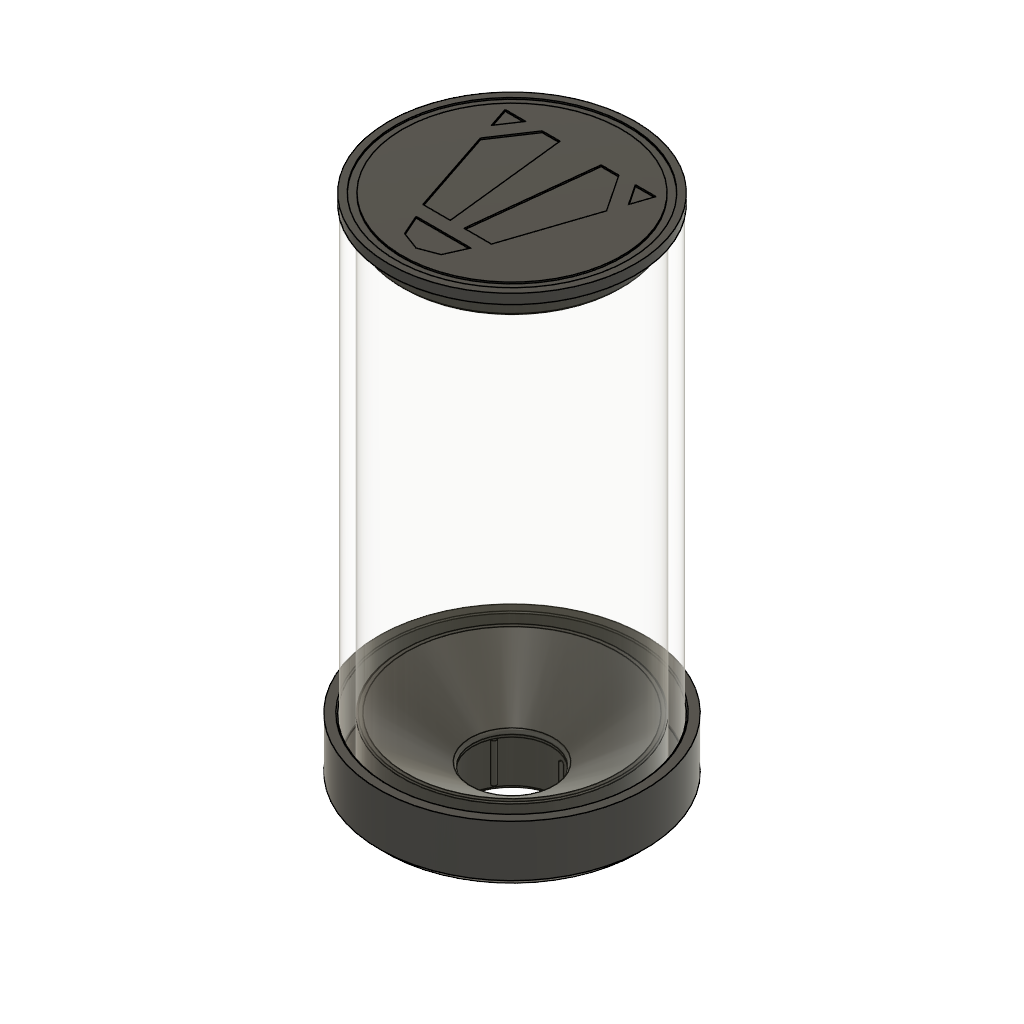
Trickler (Autodesk Fusion 360 archive; units mm, degrees)
design "PowderContainer"
part number: 2026-04-14-16-20-41-609
Autodesk Fusion 360 part; units mm, degrees
note: some values were not read from the file. Chosen so that the rebuilt part matches the saved one: how an offset face is resized. Set by a fixed rule: which sketch regions a step uses.
sketch "Sketch1" plane through (0, 0, 0) normal (0, 1, 0) x (1, 0, 0)
  circle A0 centre (0, 0) radius 25
  circle A1 centre (0, 0) radius 22.65
  dimension "d1" = 50
  dimension "d2" = 45.3
  constraint coincident A0.centre A1.centre
  measures "d1" diameter of A0
  measures "d2" diameter of A1
extrude "Extrude1" add sketch "Sketch1" along normal blind 100 makes body 1
sketch "Sketch2" plane through (0, 0, 0) normal (0, 1, 0) x (1, 0, 0)
  circle A0 centre (0, 0) radius 22.5
  circle A1 centre (0, 0) radius 25.2
  circle A2 centre (0, 0) radius 10.05
  circle A3 centre (0, 0) radius 12.05
  circle A4 centre (0, 0) radius 27.2
  circle A5 centre (0, 0) radius 8.05
  line L0 (0, -10.05) -> (8.7036, 5.025)
  line L1 (8.7036, 5.025) -> (-8.7036, 5.025)
  line L2 (-8.7036, 5.025) -> (0, -10.05)
  circle A6 centre (0, -10.05) radius 0.5
  circle A7 centre (8.7036, 5.025) radius 0.5
  circle A8 centre (-8.7036, 5.025) radius 0.5
  circle A9 centre (0, 0) radius 21
  dimension "d5" = 45
  dimension "d6" = 50.4
  dimension "d7" = 20.1
  dimension "d8" = 24.1
  dimension "d9" = 54.4
  dimension "d14" = 16.1
  dimension "d31" = 10.05
  dimension "d32" = 1
  dimension "d33" = 1
  dimension "d34" = 1
  dimension "d51" = 42
  constraint coincident A0.centre A1.centre
  constraint concentric A0 A1
  constraint concentric A1 A2
  constraint concentric A2 A3
  constraint concentric A0 A4
  constraint concentric A0 A5
  constraint coincident L0.start L2.end
  constraint coincident L0.end L1.start
  constraint coincident L1.end L2.start
  constraint concentric A2 A9
  measures "d5" diameter of A0
  measures "d6" diameter of A1
  measures "d7" diameter of A2
  measures "d8" diameter of A3
  measures "d9" diameter of A4
  measures "d14" diameter of A5
  measures "d31" distance of L0.start A0.centre
  measures "d32" diameter of A6
  measures "d33" diameter of A7
  measures "d34" diameter of A8
  measures "d51" diameter of A9
extrude "Extrude2" add sketch "Sketch2" along normal blind 10 separate body contours A0 | A2 A7 | A2 A6 | A2 A8 | A3 | A4 | A9 makes body 2 at (27.1662, 6.6667, 1.3558) makes body 3 at (22.472, 6.6667, 1.1215)
extrude "Extrude3" add sketch "Sketch2" against normal blind 2 contours A0 | A1 | A2 A7 | A2 A6 | A2 A8 | A3 | A4 | A9 bodies 2 3
extrude "Extrude4" add sketch "Sketch2" along normal blind 10 contours A2 A5 L0 A6 A7 | A2 L0 A7 | A2 L0 A6 | A2 L1 A7 | L0 L1 A7 | A5 L0 L1 A7 | L0 L2 A6 | A2 L2 A6 | A5 L0 L2 A6 | A2 A5 L1 A7 A8 | A2 A5 L2 A6 A8 | A2 L1 A8 | A2 L2 A8 | L1 L2 A8 | A5 L1 L2 A8 bodies 2
extrude "Extrude5" add sketch "Sketch2" against normal blind 11 contours A2 A7 | A2 A6 | A2 A8 | A3 bodies 2
chamfer "Chamfer4" distance 0.25 angle 45 2 edges at (-20.9774, 10, 8.1363) (-23.4946, 10, -9.1127) on bodies 2
chamfer "Chamfer5" distance 1.5 angle 45 1 edges at (-25.3593, -2, -9.8359) on bodies 2
chamfer "Chamfer6" distance 2 distance2 9 1 edges at (-11.2345, -2, 4.3575) measured on face at (21.0095, -2, 1.8754) on bodies 2
chamfer "Chamfer7" distance 1.5 angle 45 1 edges at (-13.0992, -2, -5.0807) on bodies 2
chamfer "Chamfer8" distance 13.5 distance2 9 1 edges at (-7.5052, 10, -2.911) measured on face at (17.4039, 10, 1.5053) on bodies 2
chamfer "Chamfer9" distance 0.5 distance2 0.5 1 edges at (-9.3699, 0, 3.6342) measured on face at (10.0375, -7.3333, 0.501) on bodies 2
extrude "Extrude7" add sketch "Sketch2" along normal blind -10 and the other way blind 1 contours A2 L0 A7 | A2 L0 A6 | A2 L1 A7 | L0 L1 A7 | L0 L2 A6 | A2 L2 A6 | A2 L1 A8 | A2 L2 A8 | L1 L2 A8 bodies 2
chamfer "Chamfer10" distance 0.5 angle 45 6 edges at (-8.2705, -1, -4.775) (-8.2705, -10, -4.775) (8.2705, -10, -4.775) (8.2705, -1, -4.775) (0, -1, 9.55) (0, -10, 9.55) on bodies 2
fillet "Fillet1" radius 1 1 edges at (-7.5052, 1, -2.911) on bodies 2
chamfer "Chamfer11" distance 1 angle 45 1 edges at (-9.3699, -11, 3.6342) on bodies 2
extrude "Extrude8" add sketch "Sketch2" along normal blind 100 and the other way blind -102 separate body contours A0 | A1 | A2 A5 L0 A6 A7 | A2 L0 A7 | A2 A7 | A2 A6 | A2 L0 A6 | A2 L1 A7 | L0 L1 A7 | A5 L0 L1 A7 | L0 L2 A6 | A2 L2 A6 | A5 L0 L2 A6 | A2 A5 L1 A7 A8 | A5 L0 L1 L2 | A5 L0 | A2 A5 L2 A6 A8 | A2 L1 A8 | A2 A8 | A5 L1 | A2 L2 A8 | A5 L2 | L1 L2 A8 | A5 L1 L2 A8 | A3 | A9 makes body 4
extrude "Extrude9" add sketch "Sketch2" along normal blind 100 and the other way blind -96 contours A0 bodies 4
chamfer "Chamfer12" distance 0.5 angle 45 1 edges at (-20.9774, 96, 8.1363) on bodies 4
sketch "Sketch3" plane through (0, 0, 0) normal (0, 0, 1) x (1, 0, 0)
  line L0 (0, 0) -> (0, -11)
  line L1 (0.5, -11) -> (-0.5, -11)
  line L2 (-0.5, -11) -> (-0.5, 0)
  line L3 (-0.5, 0) -> (0.5, 0)
  line L4 (0.5, 0) -> (0.5, -11)
  line L5 (0.5, -11) -> (-0.5, 0) construction
  line L6 (-0.5, -11) -> (0.5, 0) construction
  line L7 (0, 0) -> (0, -4)
  circle A0 centre (0, -4) radius 0.5
  point P0 (0, -5.5)
  dimension "d61" = 11
  dimension "d62" = 1
  dimension "d63" = 11
  dimension "d64" = 4
  dimension "d65" = 1
  constraint coincident L0.start L7.start
  constraint vertical L0
  constraint horizontal L1
  constraint perpendicular L1 L2
  constraint parallel L1 L3
  constraint parallel L2 L4
  constraint coincident L5 P0
  constraint coincident L6 P0
  constraint midpoint L0 P0
  constraint perpendicular L3 L7
  constraint coincident L7.end A0.centre
  measures "d61" distance of L0.start L0.end
  measures "d62" distance of L2.end L3.end
  measures "d63" distance of L1.end L2.end
  measures "d64" distance of L0.start L7.end
  measures "d65" diameter of A0
extrude "Extrude10" cut sketch "Sketch3" against normal blind 26 contours L0 L7 A0 | L0 L7 A0 | L0 L1 L4 A0 | L0 L1 L2 A0 bodies 2
sketch "Logo" plane through (0, 102, 0) normal (0, 1, 0) x (1, 0, 0)
  line L0 (-7.8348, 14) -> (-10.2703, 10.3468)
  line L1 (-1.4, -11.2) -> (-4.2, 14)
  line L2 (-12.8783, 6.4348) -> (-7, -11.2)
  line L3 (-4.2, 14) -> (-7.8348, 14)
  line L4 (-7, -11.2) -> (-1.4, -11.2)
  line L5 (-10.2703, 10.3468) -> (-12.8783, 6.4348)
  line L6 (7.8348, 14) -> (4.2, 14)
  line L7 (12.8783, 6.4348) -> (10.2703, 10.3468)
  line L8 (1.4, -11.2) -> (7, -11.2)
  line L9 (4.2, 14) -> (1.4, -11.2)
  line L10 (10.2703, 10.3468) -> (7.8348, 14)
  line L11 (7, -11.2) -> (12.8783, 6.4348)
  line L12 (5.6, -14) -> (3.7333, -18.2)
  line L13 (-3.7333, -18.2) -> (-5.6, -14)
  line L14 (0, -19.6) -> (-3.7333, -18.2)
  line L15 (-5.6, -14) -> (5.6, -14)
  line L16 (3.7333, -18.2) -> (0, -19.6)
  circle A0 centre (0, 0) radius 22.4
  circle A1 centre (0, 0) radius 23.8
  line L17 (-14, 9.8) -> (-15.4, 14)
  line L18 (-15.4, 14) -> (-11.2, 14)
  line L19 (-11.2, 14) -> (-14, 9.8)
  line L20 (14, 9.8) -> (11.2, 14)
  line L21 (11.2, 14) -> (15.4, 14)
  line L22 (15.4, 14) -> (14, 9.8)
scale "Scale1" [no effect]
extrude "Extrude11" cut sketch "Logo" against normal blind 0.3 bodies 4
equation "d2 = d1 - ( ( 2.35 * 2 ) * 1 mm )"
equation "d5 = d2 - 0.3 mm"
equation "d6 = d1 + 0.40 mm"
equation "d8 = d7 + 4 mm"
equation "d9 = d6 + 4 mm"
equation "d14 = d7 - 4 mm"
equation "d31 = d7 / 2"
equation "d33 = d32"
equation "d34 = d32"
equation "d51 = d5 - 3 mm"
equation "d63 = d61"
equation "d65 = d62"
named bodies: "Acrylic Pipe", "ReservoirAdapter", "ReservoirCap"

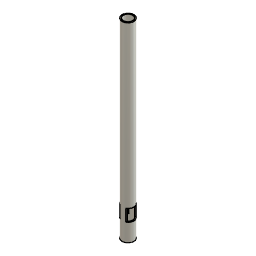
design "Pipe"
part number: 2026-04-14-16-00-10-104
Autodesk Fusion 360 part; units mm, degrees
sketch "Sketch1" plane through (0, 0, 0) normal (0, 1, 0) x (1, 0, 0)
  circle A0 centre (0, 0) radius 5
  circle A1 centre (0, 0) radius 4
  dimension "d1" = 10
  dimension "d2" = 8
  constraint coincident A0.centre A1.centre
  measures "d1" diameter of A0
  measures "d2" diameter of A1
extrude "Extrude1" add sketch "Sketch1" along normal blind 160
sketch "Sketch2" plane through (0, 0, 0) normal (0, 0, 1) x (1, 0, 0)
  line L0 (-5, 0) -> (5, 0)
  line L1 (5, 0) -> (5, 15)
  line L2 (5, 15) -> (-5, 15)
  line L3 (-5, 15) -> (-5, 0)
  line L4 (-5, 15) -> (5, 15)
  line L5 (5, 15) -> (5, 25)
  line L6 (5, 25) -> (-5, 25)
  line L7 (-5, 25) -> (-5, 15)
  line L8 (-5, 25) -> (-2.5, 25)
  line L9 (-2.5, 25) -> (-2.5, 15)
  line L10 (-2.5, 15) -> (-5, 15)
  line L11 (-5, 15) -> (-5, 25)
  line L12 (5, 15) -> (2.5, 15)
  line L13 (2.5, 15) -> (2.5, 25)
  line L14 (2.5, 25) -> (5, 25)
  line L15 (5, 25) -> (5, 15)
  dimension "d5" = 10
  dimension "d6" = 15
  dimension "d7" = 10
  dimension "d8" = 10
  dimension "d9" = 2.5
  dimension "d10" = 10
  dimension "d11" = 2.5
  dimension "d12" = 10
  constraint horizontal L0
  constraint vertical L1
  constraint horizontal L2
  constraint vertical L3
  constraint horizontal L4
  constraint vertical L5
  constraint horizontal L6
  constraint vertical L7
  constraint horizontal L8
  constraint vertical L9
  constraint horizontal L10
  constraint vertical L11
  constraint horizontal L12
  constraint vertical L13
  constraint horizontal L14
  constraint vertical L15
  measures "d5" distance of L0.start L0.end
  measures "d6" distance of L0.start L2.end
  measures "d7" distance of L2.end L1.end
  measures "d8" distance of L2.end L6.end
  measures "d9" distance of L6.end L8.end
  measures "d10" distance of L6.end L2.end
  measures "d11" distance of L1.end L12.end
  measures "d12" distance of L1.end L5.end
extrude "Extrude2" cut sketch "Sketch2" along normal mid plane 20 contours L2 L4 L6 L7 L8 L9 L10 L11 | L2 L4 L5 L6 L12 L13 L14 L15
equation "d2 = d1 - 2 mm"
equation "d5 = d1"
equation "d7 = d1"
equation "d9 = d1 / 4"
equation "d10 = d1"
equation "d11 = d1 / 4"
equation "d12 = d1"
equation "d13 = d1"
named bodies: "Pipe"

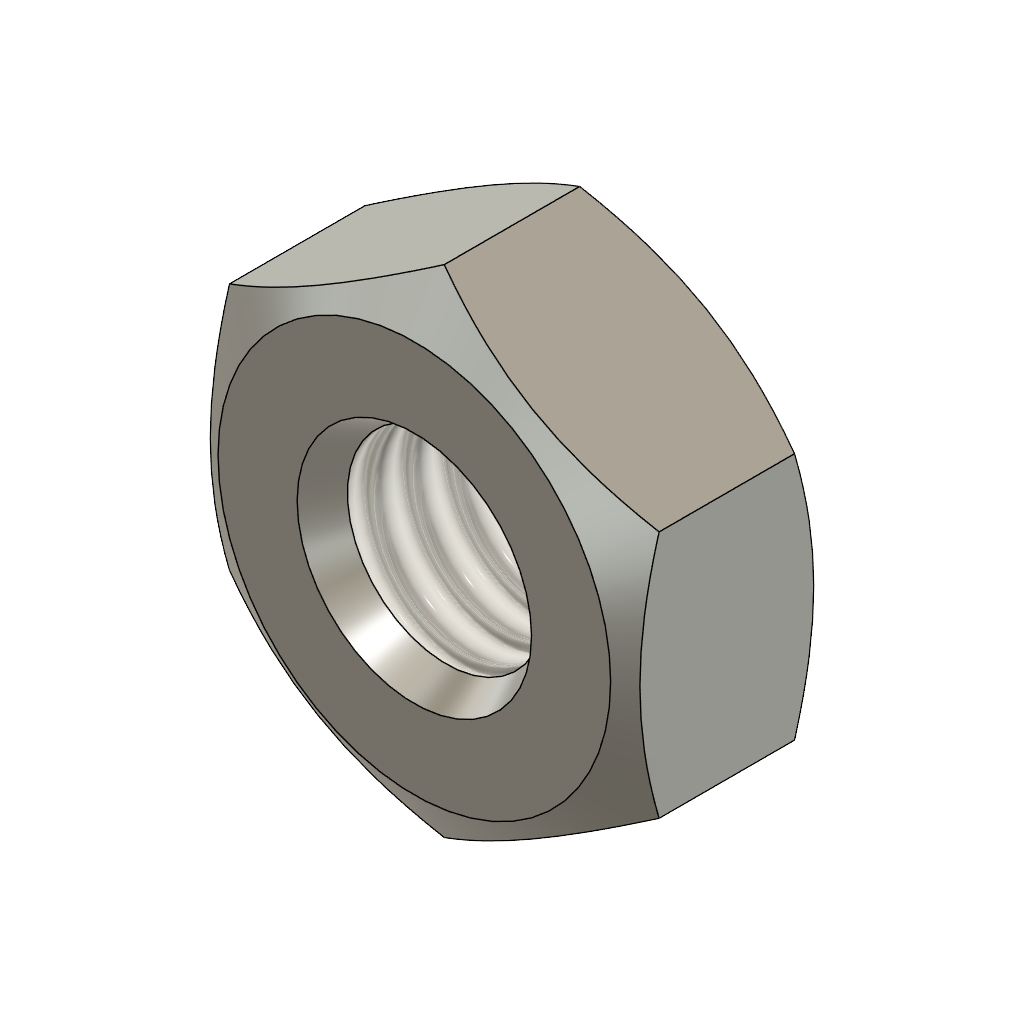
design "Hexagon Nut DIN EN 14399-4 - M3 Steel 6 Plain"
description: Hexagon Nut DIN EN 14399-4 - M3
part number: DIN EN 14399-4 - M3 Steel 6 Plain
Autodesk Fusion 360 part; units mm, degrees
sketch "Sketch1" plane through (0, 0, 0) normal (0, 1, 0) x (1, 0, 0)
  line L0 (0, 0) -> (0, -2.5)
  line L1 (-1.5, 0) -> (-2.5125, 0)
  line L2 (-2.5125, 0) -> (-3.1762, -0.3832)
  line L3 (-3.1762, -0.3832) -> (-3.1762, -2.1168)
  line L4 (-3.1762, -2.1168) -> (-2.5125, -2.5)
  line L5 (-2.5125, -2.5) -> (-1.5, -2.5)
  line L6 (-1.5, -2.5) -> (-1.5, 0)
  dimension "d121" = 3
  dimension "d122" = 30
  dimension "d123" = 30
  dimension "d128" = 6.3525
  dimension "d172" = 5.025
  dimension "d179" = 2.5
  constraint vertical L0
  constraint coincident L0 L0.end
  constraint coincident origin L0
  constraint horizontal L1
  constraint coincident L0.start L1
  constraint coincident L0.start origin
  constraint coincident L0.end L5
  constraint vertical L1.end L4.end
  measures "d122" angle of L1 L2
  measures "d123" angle of L4 L5
  measures "d179" distance of L1 L5
revolve "Revolve1" add sketch "Sketch1" angle 360 about axis through (0, 0, 0) along (0, 0, 1)
sketch "Sketch8" plane through (0, 0, 2.5) normal (0, 0, 1) x (1, 0, 0)
  line L0 (-2.75, -1.5894) -> (-2.75, 1.5894)
  circle A0 centre (0, 0) radius 1.5
  circle A1 centre (0, 0) radius 3.1762
  dimension "d114" = 2.75
  constraint coincident L0.end A1
  constraint coincident L0.start A1
  constraint vertical L0
  measures "d114" distance of A0.centre L0
extrude "Extrude5" cut sketch "Sketch8" against normal blind 2.5 contours L0 A1 picked at (-2.8188, -0.3871)
pattern_circular "C-Pattern2" count 6 over 360 about axis through (0, 0, 1.75) along (0, 0, 1) of "Extrude5"
thread "Thread3" "ISO Metric profile 3.0 M3x0.5 M3x0.5 6H" major diameter 3.086 minor diameter 2.529 pitch 0.5 angle 60 resizes the face on face at (-1.4981, 0.0748, 1.6667)
sketch "Sketch12" plane through (0, 0, 0) normal (0, 1, 0) x (1, 0, 0)
  line L0 (-1.5, 0) -> (0, 0)
  line L1 (-0.7783, -1.25) -> (-1.5, 0)
  line L2 (-1.5, -2.5) -> (0, -2.5)
  line L3 (-0.7783, -1.25) -> (-1.5, -2.5)
  line L4 (0, 0) -> (0, -2.5)
  dimension "d169" = 60
  dimension "d177" = 1.5
  dimension "d178" = 60
  constraint horizontal L0
  constraint coincident L1.start L3.start
  constraint vertical L0.start L2.start
  constraint coincident L2.end L4.end
  constraint coincident L0.end L4.start
  constraint perpendicular L2 L4
  measures "d169" angle of L2 L3
  measures "d177" distance of L0.start L4
  measures "d178" angle of L0 L1
revolve "Revolve3" cut sketch "Sketch12" angle 360 about axis through (0, 0, 1.75) along (0, 0, 1)
equation "adsk_nheig = 2.50 mm"
equation "adsk_maxdia = 6.3525 mm"
equation "adsk_nomdia = 3.00 mm"
equation "d89 = -adsk_nheig"
equation "adsk_waflat = 5.50 mm"
equation "d114 = adsk_waflat / 2"
equation "adsk_chamang1 = 30.00 deg"
equation "adsk_chamang2 = 30.00 deg"
equation "d121 = adsk_nomdia"
equation "d122 = adsk_chamang1"
equation "d123 = adsk_chamang2"
equation "d128 = adsk_maxdia"
equation "d163 = adsk_nheig"
equation "adsk_beardia = 5.025 mm"
equation "d172 = adsk_beardia"
equation "d177 = adsk_nomdia * 0.5"
equation "d179 = adsk_nheig"

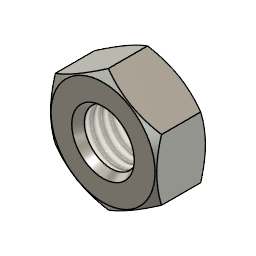
design "Hexagon Nut DIN 934 - M10 x 1.5 Steel 6 Plain"
description: Hexagon Nut DIN 934 - M10 x 1.5
part number: DIN 934 - M10 x 1.5 Steel 6 Plain
Autodesk Fusion 360 part; units mm, degrees
sketch "Sketch1" plane through (0, 0, 0) normal (0, 1, 0) x (1, 0, 0)
  line L0 (0, 0) -> (0, -8)
  line L1 (-5, 0) -> (-8.33, 0)
  line L2 (-8.33, 0) -> (-9.8175, -0.8588)
  line L3 (-9.8175, -0.8588) -> (-9.8175, -7.1412)
  line L4 (-9.8175, -7.1412) -> (-8.33, -8)
  line L5 (-8.33, -8) -> (-5, -8)
  line L6 (-5, -8) -> (-5, 0)
  dimension "d121" = 10
  dimension "d122" = 30
  dimension "d123" = 30
  dimension "d128" = 19.635
  dimension "d172" = 16.66
  dimension "d179" = 8
  constraint vertical L0
  constraint coincident L0 L0.end
  constraint coincident origin L0
  constraint horizontal L1
  constraint coincident L0.start L1
  constraint coincident L0.start origin
  constraint coincident L0.end L5
  constraint vertical L1.end L4.end
  measures "d122" angle of L1 L2
  measures "d123" angle of L4 L5
  measures "d179" distance of L1 L5
revolve "Revolve1" add sketch "Sketch1" angle 360 about axis through (0, 0, 0) along (0, 0, 1)
sketch "Sketch8" plane through (0, 0, 8) normal (0, 0, 1) x (1, 0, 0)
  line L0 (-8.5, -4.9126) -> (-8.5, 4.9126)
  circle A0 centre (0, 0) radius 5
  circle A1 centre (0, 0) radius 9.8175
  dimension "d114" = 8.5
  constraint coincident L0.end A1
  constraint coincident L0.start A1
  constraint vertical L0
  measures "d114" distance of A0.centre L0
extrude "Extrude5" cut sketch "Sketch8" against normal blind 8 contours L0 A1 picked at (-8.7126, 1.1966)
pattern_circular "C-Pattern2" count 6 over 360 about axis through (0, 0, 1.75) along (0, 0, 1) of "Extrude5"
thread "Thread3" "ISO Metric profile 10.0 M10x1.5 M10x1.5 6H" major diameter 10.198 minor diameter 8.526 pitch 1.5 angle 60 resizes the face on face at (-4.9752, 0.4978, 5.3333)
sketch "Sketch12" plane through (0, 0, 0) normal (0, 1, 0) x (1, 0, 0)
  line L0 (-5, 0) -> (0, 0)
  line L1 (-2.6906, -4) -> (-5, 0)
  line L2 (-5, -8) -> (0, -8)
  line L3 (-2.6906, -4) -> (-5, -8)
  line L4 (0, 0) -> (0, -8)
  dimension "d169" = 60
  dimension "d177" = 5
  dimension "d178" = 60
  constraint horizontal L0
  constraint coincident L1.start L3.start
  constraint vertical L0.start L2.start
  constraint coincident L2.end L4.end
  constraint coincident L0.end L4.start
  constraint perpendicular L2 L4
  measures "d169" angle of L2 L3
  measures "d177" distance of L0.start L4
  measures "d178" angle of L0 L1
revolve "Revolve3" cut sketch "Sketch12" angle 360 about axis through (0, 0, 1.75) along (0, 0, 1)
equation "adsk_nheig = 8.00 mm"
equation "adsk_maxdia = 19.635 mm"
equation "adsk_nomdia = 10.00 mm"
equation "d89 = -adsk_nheig"
equation "adsk_waflat = 17.00 mm"
equation "d114 = adsk_waflat / 2"
equation "adsk_chamang1 = 30.00 deg"
equation "adsk_chamang2 = 30.00 deg"
equation "d121 = adsk_nomdia"
equation "d122 = adsk_chamang1"
equation "d123 = adsk_chamang2"
equation "d128 = adsk_maxdia"
equation "d163 = adsk_nheig"
equation "adsk_beardia = adsk_waflat * 0.98"
equation "d172 = adsk_beardia"
equation "d177 = adsk_nomdia * 0.5"
equation "d179 = adsk_nheig"
